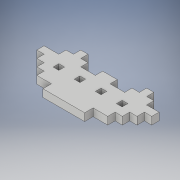
# Autodesk Inventor part: Monster1
Saved by Autodesk Inventor 2019 (Build 230136000, 136)
## iProperties
Created: 2018-12-03
Part Number: Monster1
Material: Generic
Document SubType Name: Modeling
Designer: Administrator
Density: 1 g/cm^3
Appearance: Default
Author: Administrator
Autodesk Inventor part; units mm, degrees
ref_plane "YZ Plane" through (0, 0, 0) normal (1, 0, 0) x (0, 1, 0)
ref_plane "XZ Plane" through (0, 0, 0) normal (0, 1, 0) x (-1, 0, 0)
ref_plane "XY Plane" through (0, 0, 0) normal (0, 0, 1) x (1, 0, 0)
sketch "Sketch1" plane through (0, 0, 0) normal (0, 1, 0) x (-1, 0, 0)
  line L0 (0, 0) -> (326.2264, 0) construction
  line L1 (326.2264, 0) -> (326.2264, -146.0251) construction
  line L2 (326.2264, -146.0251) -> (0, -146.0251) construction
  line L3 (0, -146.0251) -> (0, 0) construction
  line L4 (67.2736, -57.5928) -> (73.4159, -57.5928)
  line L5 (73.4159, -57.5928) -> (73.4159, -51.4505)
  line L6 (73.4159, -51.4505) -> (85.7005, -51.4505)
  line L7 (85.7005, -51.4505) -> (85.7005, -57.5928)
  line L8 (85.7005, -57.5928) -> (91.8428, -57.5928)
  line L9 (91.8428, -57.5928) -> (91.8428, -63.7351)
  line L10 (91.8428, -63.7351) -> (97.9851, -63.7351)
  line L11 (97.9851, -63.7351) -> (97.9851, -57.5928)
  line L12 (97.9851, -57.5928) -> (104.1274, -57.5928)
  line L13 (104.1274, -57.5928) -> (104.1274, -51.4505)
  line L14 (104.1274, -51.4505) -> (116.412, -51.4505)
  line L15 (116.412, -51.4505) -> (116.412, -45.3082)
  line L16 (116.412, -45.3082) -> (110.2697, -45.3082)
  line L17 (110.2697, -45.3082) -> (110.2697, -39.1659)
  line L18 (110.2697, -39.1659) -> (104.1274, -39.1659)
  line L19 (104.1274, -39.1659) -> (104.1274, -33.0236)
  line L20 (104.1274, -33.0236) -> (97.9851, -33.0236)
  line L21 (97.9851, -33.0236) -> (97.9851, -26.8813)
  line L22 (97.9851, -26.8813) -> (85.7005, -26.8813)
  line L23 (85.7005, -26.8813) -> (85.7005, -20.739)
  line L24 (69.1807, -19.7772) -> (85.7005, -19.7772)
  line L25 (85.7005, -19.7772) -> (85.7005, -20.739)
  line L26 (67.2736, -57.5928) -> (61.1313, -57.5928)
  line L27 (61.1313, -57.5928) -> (61.1313, -51.4505)
  line L28 (61.1313, -51.4505) -> (48.8467, -51.4505)
  line L29 (48.8467, -51.4505) -> (48.8467, -57.5928)
  line L30 (48.8467, -57.5928) -> (42.7043, -57.5928)
  line L31 (42.7043, -57.5928) -> (42.7043, -63.7351)
  line L32 (42.7043, -63.7351) -> (36.562, -63.7351)
  line L33 (36.562, -63.7351) -> (36.562, -57.5928)
  line L34 (36.562, -57.5928) -> (30.4197, -57.5928)
  line L35 (30.4197, -57.5928) -> (30.4197, -51.4505)
  line L36 (30.4197, -51.4505) -> (20.0422, -51.4505)
  line L37 (20.0422, -51.4505) -> (20.0422, -45.3082)
  line L38 (20.0422, -45.3082) -> (26.1845, -45.3082)
  line L39 (26.1845, -45.3082) -> (26.1845, -39.1659)
  line L40 (26.1845, -39.1659) -> (32.3268, -39.1659)
  line L41 (32.3268, -39.1659) -> (32.3268, -33.0236)
  line L42 (32.3268, -33.0236) -> (38.4691, -33.0236)
  line L43 (38.4691, -33.0236) -> (38.4691, -26.8813)
  line L44 (38.4691, -26.8813) -> (50.7538, -26.8813)
  line L45 (50.7538, -26.8813) -> (50.7538, -20.739)
  line L46 (69.1807, -19.7772) -> (50.7538, -19.7772)
  line L47 (50.7538, -19.7772) -> (50.7538, -20.739)
  line L48 (39.2885, -39.7662) -> (39.2885, -44.5453)
  line L49 (39.2885, -44.5453) -> (44.0675, -44.5453)
  line L50 (44.0675, -44.5453) -> (44.0675, -39.7662)
  line L51 (44.0675, -39.7662) -> (39.2885, -39.7662)
  line L52 (56.9879, -39.7662) -> (56.9879, -44.5453)
  line L53 (56.9879, -44.5453) -> (61.7669, -44.5453)
  line L54 (56.9879, -39.7662) -> (61.7669, -39.7662)
  line L55 (61.7669, -39.7662) -> (61.7669, -44.5453)
  line L56 (74.6873, -39.7662) -> (79.4663, -39.7662)
  line L57 (79.4663, -39.7662) -> (79.4663, -44.5453)
  line L58 (79.4663, -44.5453) -> (74.6873, -44.5453)
  line L59 (74.6873, -44.5453) -> (74.6873, -39.7662)
  line L60 (92.3867, -39.7662) -> (97.1657, -39.7662)
  line L61 (97.1657, -39.7662) -> (97.1657, -44.5453)
  line L62 (97.1657, -44.5453) -> (92.3867, -44.5453)
  line L63 (92.3867, -44.5453) -> (92.3867, -39.7662)
  dimension "d3" = 6.1423
  dimension "d6" = 6.1423
  dimension "d7" = 6.1423
  dimension "d8" = 6.1423
  dimension "d9" = 6.1423
  dimension "d10" = 6.1423
  dimension "d11" = 6.1423
  dimension "d12" = 6.1423
  dimension "d13" = 12.2846
  dimension "d14" = 12.2846
  dimension "d15" = 6.1423
  dimension "d16" = 6.1423
  dimension "d17" = 6.1423
  dimension "d18" = 6.1423
  dimension "d19" = 6.1423
  dimension "d20" = 12.2846
  dimension "d21" = 6.1423
  dimension "d22" = 6.1423
  dimension "d23" = 6.1423
  dimension "d29" = 12.9204
  dimension "d30" = 12.9204
  dimension "d31" = 13.104
  dimension "d32" = 13.104
  dimension "d33" = 12.9204
  dimension "d34" = 4.779
  dimension "d35" = 4.779
  dimension "d36" = 4.779
  dimension "d37" = 4.779
  dimension "d38" = 4.779
  dimension "d39" = 4.779
  dimension "d40" = 4.779
  constraints: 120 end point, 24 perpendicular, 21 point on line, 3 vertical, 1 horizontal, 2 other
  measures "d3" distance of L19.end L20.end
  measures "d6" distance of L20.end L21.end
  measures "d7" distance of L18.end L19.end
  measures "d8" distance of L17.end L18.end
  measures "d9" distance of L15.end L16.end
  measures "d10" distance of L16.end L17.end
  measures "d11" distance of L14.end L15.end
  measures "d12" distance of L22.end L23.end
  measures "d13" distance of L21.end L22.end
  measures "d14" distance of L13.end L14.end
  measures "d15" distance of L11.end L12.end
  measures "d16" distance of L12.end L13.end
  measures "d17" distance of L10.end L11.end
  measures "d18" distance of L9.end L10.end
  measures "d19" distance of L7.end L8.end
  measures "d20" distance of L5.end L6.end
  measures "d21" distance of L4.end L5.end
  measures "d22" distance of L6.end L7.end
  measures "d23" distance of L4.start L4.end
  measures "d29" distance between parallel lines of L63 L57
  measures "d30" distance between parallel lines of L59 L55
  measures "d31" distance between parallel lines of L17 L61
  measures "d32" distance between parallel lines of L39 L48
  measures "d33" distance between parallel lines of L52 L50
  measures "d34" distance between parallel lines of L49 L51
  measures "d35" distance between parallel lines of L50 L48
  measures "d36" distance of L52.start L52.end
  measures "d37" distance of L52.end L53.end
  measures "d38" distance of L56.start L56.end
  measures "d39" distance between parallel lines of L57 L59
  measures "d40" distance of L60.start L60.end
extrude "Extrusion1" add sketch "Sketch1" along normal blind 6.35
equation "\"d6\" = d3"
equation "\"d7\" = d6"
equation "\"d8\" = d3"
equation "\"d9\" = d7"
equation "\"d10\" = d7"
equation "\"d11\" = d10"
equation "\"d12\" = d6"
equation "\"d13\" = 2 * d3"
equation "\"d14\" = d13"
equation "\"d15\" = d6"
equation "\"d16\" = d11"
equation "\"d17\" = d16"
equation "\"d18\" = d17"
equation "\"d19\" = d17"
equation "\"d20\" = d13"
equation "\"d23\" = 0.5 * d13"
equation "\"d30\" = d29"
equation "\"d32\" = d31"
equation "\"d33\" = d30"
equation "\"d35\" = d34"
equation "\"d37\" = d35"
equation "\"d38\" = d36"
equation "\"d40\" = d38"
body "Solid1"
